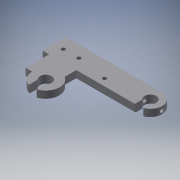
# Autodesk Inventor part: Hand - Digit 0-1
Saved by Autodesk Inventor 2017 (Build 210142000, 142)
## iProperties
Created: 2016-09-27
Part Number: Hand - Digit 0-1
Material: Generic
Document SubType Name: Modeling
Designer: cmcdona
Density: 1 g/cm^3
Appearance: Default
Author: cmcdona
Autodesk Inventor part; units mm, degrees
ref_plane "YZ Plane" through (0, 0, 0) normal (1, 0, 0) x (0, 1, 0)
ref_plane "XZ Plane" through (0, 0, 0) normal (0, 1, 0) x (-1, 0, 0)
ref_plane "XY Plane" through (0, 0, 0) normal (0, 0, 1) x (1, 0, 0)
sketch "Sketch1" plane through (0, 0, 0) normal (0, 0, 1) x (1, 0, 0)
  line L0 (0, 0) -> (5, 0)
  line L1 (5, 0) -> (5, -18)
  line L2 (5, -18) -> (26, -18)
  line L3 (26, -18) -> (26, 0)
  line L4 (26, 0) -> (74, 0)
  arc A0 (74, 0) -> (74, 18) centre (74, 9) ccw
  line L5 (74, 18) -> (0, 18)
  line L6 (0, 18) -> (0, 0)
  circle A1 centre (20.5, -18) radius 10.5
  dimension "d0" = 5
  dimension "d1" = 18
  dimension "d2" = 21
  dimension "d3" = 18
  dimension "d4" = 48
  dimension "d5" = 18
  dimension "d6" = 9
  dimension "d7" = 74
  dimension "d8" = 21
  constraints: 14 end point, 3 perpendicular, 3 point on line, 2 centre point, 2 horizontal, 2 point on circle
  measures "d0" distance of L0.start L0.end
  measures "d1" distance of L0.end L1.end
  measures "d2" distance of L1.end L2.end
  measures "d3" distance of L2.end L3.end
  measures "d4" distance of L3.end L4.end
  measures "d5" distance of L4.end L5.start
  measures "d6" radius of A0
  measures "d7" distance of L5.start L5.end
  measures "d8" diameter of A1
extrude "Extrusion1" add sketch "Sketch1" along normal blind 6
sketch "Sketch2" plane through (0, 0, 0) normal (0, 0, -1) x (-1, 0, 0)
  circle A0 centre (-74, 9) radius 4.5
  arc A1 (-26, -9.0557) -> (-10, -18) centre (-20.5, -18) ccw projected
  circle A2 centre (-20.5, -18) radius 4.5
  point P0 (0, 0)
  dimension "d11" = 9
  dimension "d12" = 9
  constraints: 2 centre point, 1 coincident
  measures "d11" diameter of A0
  measures "d12" diameter of A2
extrude "Extrusion2" cut sketch "Sketch2" against normal through all
sketch "Sketch3" plane through (0, 0, 0) normal (0, 0, -1) x (-1, 0, 0)
  circle A0 centre (-7, 9) radius 1.5
  circle A1 centre (-19, 9) radius 1.5
  point P0 (0, 0)
  dimension "d16" = 3
  dimension "d17" = 3
  constraints: 2 centre point
  measures "d16" diameter of A0
  measures "d17" diameter of A1
extrude "Extrusion3" cut sketch "Sketch3" against normal through all
ref_plane "Work Plane1" through (83, 0, 0) normal (-1, 0, 0) x (0, 0, 1)
sketch "Sketch4" plane through (83, 0, 0) normal (-1, 0, 0) x (0, 0, 1)
  circle A0 centre (3, 9) radius 1.5
  point P0 (0, 0)
  dimension "d22" = 3
  constraints: 1 centre point
  measures "d22" diameter of A0
extrude "Extrusion4" cut sketch "Sketch4" along normal blind 18
fillet "Fillet3" radius 1 8 edges at (83, 9, 0) (50, 0, 0) (37, 18, 0) (2.5, 0, 0) (5, -9, 0) (25.6235, -27.1652, 0) (7.5, -18, 0) (26, -4.5279, 0)
sketch "Sketch5" plane through (0, 18, 6) normal (0, 1, 0) x (1, 0, 0)
  circle A0 centre (69, 2.5) radius 1.5
  circle A1 centre (58, 2.5) radius 1.5
  point P0 (0, 6)
  dimension "d26" = 3
  dimension "d27" = 3
  constraints: 2 centre point
  measures "d26" diameter of A0
  measures "d27" diameter of A1
extrude "Extrusion5" cut sketch "Sketch5" against normal blind 5
sketch "Sketch6" plane through (0, 0, 6) normal (0, 0, 1) x (1, 0, 0)
  line L0 (71, 0) -> (77, 0)
  line L1 (77, 0) -> (77, 6)
  line L2 (77, 6) -> (71, 6)
  line L3 (71, 6) -> (71, 0)
  line L4 (17.5, -18) -> (23.5, -18)
  line L5 (23.5, -18) -> (23.5, -29)
  line L6 (23.5, -29) -> (17.5, -29)
  line L7 (17.5, -29) -> (17.5, -18)
  point P0 (0, 0)
  dimension "d30" = 6
  dimension "d31" = 6
  dimension "d32" = 6
  dimension "d33" = 11
  constraints: 16 end point, 4 parallel, 2 horizontal, 2 perpendicular
  measures "d30" distance of L2.end L1.end
  measures "d31" distance of L1.end L0.end
  measures "d32" distance of L5.end L6.end
  measures "d33" distance of L4.end L5.end
extrude "Extrusion6" cut sketch "Sketch6" against normal through all
sketch "Sketch7" plane through (0, 0, 0) normal (0, 0, -1) x (-1, 0, 0)
  arc A0 (-38.7148, 11.0023) -> (-38.2652, 13.3358) centre (-45.6076, 13.5402) ccw projected
  arc A1 (-38.1755, 10.6175) -> (-38.7148, 11.0023) centre (-42.3608, 5.3217) ccw projected
  arc A2 (-36.1152, 11.8018) -> (-38.1755, 10.6175) centre (-33.5331, 4.9255) ccw projected
  arc A3 (-35.5101, 11.1585) -> (-36.1152, 11.8018) centre (-42.3608, 5.3217) ccw projected
  arc A4 (-36.8185, 9.1746) -> (-35.5101, 11.1585) centre (-42.2153, 14.1571) ccw projected
  arc A5 (-36.4675, 8.6128) -> (-36.8185, 9.1746) centre (-42.3608, 5.3217) ccw projected
  arc A6 (-34.1108, 8.9185) -> (-36.4675, 8.6128) centre (-34.3567, 1.5774) ccw projected
  arc A7 (-33.798, 8.0925) -> (-34.1108, 8.9185) centre (-42.3608, 5.3217) ccw projected
  arc A8 (-35.7659, 6.7603) -> (-33.798, 8.0925) centre (-38.8453, 13.4288) ccw projected
  arc A9 (-35.6566, 6.107) -> (-35.7659, 6.7603) centre (-42.3608, 5.3217) ccw projected
  arc A10 (-33.3623, 5.4875) -> (-35.6566, 6.107) centre (-36.3988, -1.2006) ccw projected
  arc A11 (-33.3894, 4.6047) -> (-33.3623, 5.4875) centre (-42.3608, 5.3217) ccw projected
  arc A12 (-35.7174, 4.1271) -> (-33.3894, 4.6047) centre (-36.0104, 11.4664) ccw projected
  arc A13 (-35.8664, 3.4816) -> (-35.7174, 4.1271) centre (-42.3608, 5.3217) ccw projected
  arc A14 (-33.9838, 2.0314) -> (-35.8664, 3.4816) centre (-39.3486, -2.9857) ccw projected
  arc A15 (-34.3467, 1.2261) -> (-33.9838, 2.0314) centre (-42.3608, 5.3217) ccw projected
  arc A16 (-36.6802, 1.6757) -> (-34.3467, 1.2261) centre (-34.1423, 8.5684) ccw projected
  arc A17 (-37.0649, 1.1364) -> (-36.6802, 1.6757) centre (-42.3608, 5.3217) ccw projected
  arc A18 (-35.8806, -0.9239) -> (-37.0649, 1.1364) centre (-42.757, -3.506) ccw projected
  arc A19 (-36.524, -1.529) -> (-35.8806, -0.9239) centre (-42.3608, 5.3217) ccw projected
  arc A20 (-38.5079, -0.2207) -> (-36.524, -1.529) centre (-33.5254, 5.1762) ccw projected
  arc A21 (-39.0697, -0.5716) -> (-38.5079, -0.2207) centre (-42.3608, 5.3217) ccw projected
  arc A22 (-38.764, -2.9284) -> (-39.0697, -0.5716) centre (-46.105, -2.6824) ccw projected
  arc A23 (-39.59, -3.2412) -> (-38.764, -2.9284) centre (-42.3608, 5.3217) ccw projected
  arc A24 (-40.9222, -1.2732) -> (-39.59, -3.2412) centre (-34.2536, 1.8061) ccw projected
  arc A25 (-41.5755, -1.3825) -> (-40.9222, -1.2732) centre (-42.3608, 5.3217) ccw projected
  arc A26 (-42.1949, -3.6768) -> (-41.5755, -1.3825) centre (-48.8831, -0.6403) ccw projected
  arc A27 (-43.0777, -3.6497) -> (-42.1949, -3.6768) centre (-42.3608, 5.3217) ccw projected
  arc A28 (-43.5554, -1.3218) -> (-43.0777, -3.6497) centre (-36.2161, -1.0287) ccw projected
  arc A29 (-44.2008, -1.1727) -> (-43.5554, -1.3218) centre (-42.3608, 5.3217) ccw projected
  arc A30 (-45.6511, -3.0553) -> (-44.2008, -1.1727) centre (-50.6681, 2.3095) ccw projected
  arc A31 (-46.4564, -2.6925) -> (-45.6511, -3.0553) centre (-42.3608, 5.3217) ccw projected
  arc A32 (-46.0068, -0.3589) -> (-46.4564, -2.6925) centre (-39.114, -2.8968) ccw projected
  arc A33 (-46.5461, 0.0258) -> (-46.0068, -0.3589) centre (-42.3608, 5.3217) ccw projected
  arc A34 (-48.6064, -1.1585) -> (-46.5461, 0.0258) centre (-51.1885, 5.7179) ccw projected
  arc A35 (-49.2115, -0.5151) -> (-48.6064, -1.1585) centre (-42.3608, 5.3217) ccw projected
  arc A36 (-47.9032, 1.4688) -> (-49.2115, -0.5151) centre (-42.5063, -3.5137) ccw projected
  arc A37 (-48.2541, 2.0306) -> (-47.9032, 1.4688) centre (-42.3608, 5.3217) ccw projected
  arc A38 (-50.6108, 1.7249) -> (-48.2541, 2.0306) centre (-50.3649, 9.0659) ccw projected
  arc A39 (-50.9237, 2.5508) -> (-50.6108, 1.7249) centre (-42.3608, 5.3217) ccw projected
  arc A40 (-48.9557, 3.883) -> (-50.9237, 2.5508) centre (-45.8763, -2.7855) ccw projected
  arc A41 (-49.065, 4.5364) -> (-48.9557, 3.883) centre (-42.3608, 5.3217) ccw projected
  arc A42 (-51.3593, 5.1558) -> (-49.065, 4.5364) centre (-48.3228, 11.8439) ccw projected
  arc A43 (-51.3322, 6.0386) -> (-51.3593, 5.1558) centre (-42.3608, 5.3217) ccw projected
  arc A44 (-49.0043, 6.5163) -> (-51.3322, 6.0386) centre (-48.7112, -0.823) ccw projected
  arc A45 (-48.8552, 7.1617) -> (-49.0043, 6.5163) centre (-42.3608, 5.3217) ccw projected
  arc A46 (-50.7378, 8.612) -> (-48.8552, 7.1617) centre (-45.373, 13.629) ccw projected
  arc A47 (-50.3749, 9.4172) -> (-50.7378, 8.612) centre (-42.3608, 5.3217) ccw projected
  arc A48 (-48.0414, 8.9677) -> (-50.3749, 9.4172) centre (-50.5793, 2.0749) ccw projected
  arc A49 (-47.6567, 9.5069) -> (-48.0414, 8.9677) centre (-42.3608, 5.3217) ccw projected
  arc A50 (-48.841, 11.5673) -> (-47.6567, 9.5069) centre (-41.9646, 14.1494) ccw projected
  arc A51 (-48.1976, 12.1724) -> (-48.841, 11.5673) centre (-42.3608, 5.3217) ccw projected
  arc A52 (-46.2137, 10.864) -> (-48.1976, 12.1724) centre (-51.1962, 5.4671) ccw projected
  arc A53 (-45.6519, 11.215) -> (-46.2137, 10.864) centre (-42.3608, 5.3217) ccw projected
  arc A54 (-45.9576, 13.5717) -> (-45.6519, 11.215) centre (-38.6166, 13.3258) ccw projected
  arc A55 (-45.1317, 13.8845) -> (-45.9576, 13.5717) centre (-42.3608, 5.3217) ccw projected
  arc A56 (-43.7995, 11.9166) -> (-45.1317, 13.8845) centre (-50.468, 8.8372) ccw projected
  arc A57 (-43.1461, 12.0258) -> (-43.7995, 11.9166) centre (-42.3608, 5.3217) ccw projected
  arc A58 (-42.5267, 14.3201) -> (-43.1461, 12.0258) centre (-35.8385, 11.2837) ccw projected
  arc A59 (-41.6439, 14.2931) -> (-42.5267, 14.3201) centre (-42.3608, 5.3217) ccw projected
  arc A60 (-41.1662, 11.9651) -> (-41.6439, 14.2931) centre (-48.5055, 11.6721) ccw projected
  arc A61 (-40.5208, 11.816) -> (-41.1662, 11.9651) centre (-42.3608, 5.3217) ccw projected
  arc A62 (-39.0705, 13.6987) -> (-40.5208, 11.816) centre (-34.0535, 8.3339) ccw projected
  arc A63 (-38.2652, 13.3358) -> (-39.0705, 13.6987) centre (-42.3608, 5.3217) ccw projected
  circle A64 centre (-42.3608, 5.3217) radius 1.5
  point P0 (0, 0)
  dimension "d36" = 3
  constraints: 1 centre point, 1 coincident
  measures "d36" diameter of A64
extrude "Extrusion7" cut sketch "Sketch7" against normal through all contours A64
body "Solid1"
